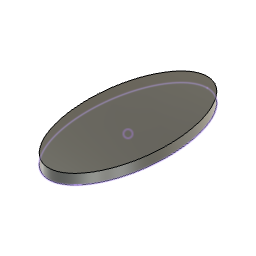
oval (Autodesk Fusion 360 design; units mm, degrees)
Autodesk Fusion 360 part; units mm, degrees
sketch "Sketch1" plane through (0, 0, 0) normal (0, 0, 1) x (1, 0, 0)
  ellipse E0 centre (0, 0) end of major axis (15, 0) minor radius 30
  line L0 (-15, 0) -> (15, 0)
  line L1 (0, -30) -> (0, 30)
  dimension "d1" = 60
  constraint coincident E0.centre origin
  constraint horizontal L0
  constraint coincident E0 L0.start
  constraint coincident E0 L0.end
  constraint coincident E0 L1.start
  constraint coincident E0 L1.end
extrude "Extrude1" add sketch "Sketch1" along normal blind 3.8
sketch "Sketch2" plane through (0, 0, 0) normal (0, 0, 1) x (1, 0, 0)
  ellipse E0 centre (0, 0) end of major axis (0, 30) minor radius 15
